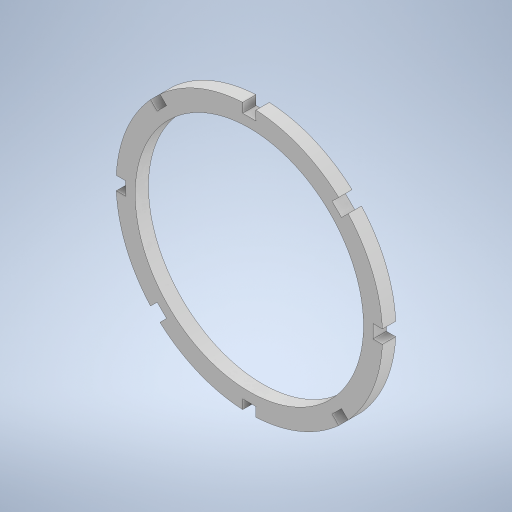
# Autodesk Inventor part: Ozji obroc
Saved by Autodesk Inventor 2023 (Build 270158000, 158)
## iProperties
Created: 2022-12-16
Part Number: Ozji obroc
Material: Generic
Document SubType Name: Modeling
Designer: David Zindović
Density: 1 g/cm^3
Appearance: Default
Author: David Zindović
Autodesk Inventor part; units mm, degrees
ref_plane "YZ Plane" through (0, 0, 0) normal (1, 0, 0) x (0, 1, 0)
ref_plane "XZ Plane" through (0, 0, 0) normal (0, 1, 0) x (-1, 0, 0)
ref_plane "XY Plane" through (0, 0, 0) normal (0, 0, 1) x (1, 0, 0)
sketch "Sketch1" plane through (0, 0, 0) normal (0, 0, 1) x (1, 0, 0)
  circle A0 centre (0, 0) radius 35
  circle A1 centre (0, 0) radius 30
  line L0 (32.5, 1.75) -> (35, 1.75)
  line L1 (35, 1.75) -> (35, -1.75)
  line L2 (35, -1.75) -> (32.5, -1.75)
  line L3 (32.5, -1.75) -> (32.5, 1.75)
  line L4 (30, 0) -> (35, 0)
  line L5 (24.2184, 21.7435) -> (21.7435, 24.2184)
  line L6 (21.7435, 24.2184) -> (23.5113, 25.9862)
  line L7 (25.9862, 23.5113) -> (24.2184, 21.7435)
  line L8 (23.5113, 25.9862) -> (25.9862, 23.5113)
  line L9 (1.75, 32.5) -> (-1.75, 32.5)
  line L10 (-1.75, 32.5) -> (-1.75, 35)
  line L11 (1.75, 35) -> (1.75, 32.5)
  line L12 (-1.75, 35) -> (1.75, 35)
  line L13 (-21.7435, 24.2184) -> (-24.2184, 21.7435)
  line L14 (-24.2184, 21.7435) -> (-25.9862, 23.5113)
  line L15 (-23.5113, 25.9862) -> (-21.7435, 24.2184)
  line L16 (-25.9862, 23.5113) -> (-23.5113, 25.9862)
  line L17 (-32.5, 1.75) -> (-32.5, -1.75)
  line L18 (-32.5, -1.75) -> (-35, -1.75)
  line L19 (-35, 1.75) -> (-32.5, 1.75)
  line L20 (-35, -1.75) -> (-35, 1.75)
  line L21 (-24.2184, -21.7435) -> (-21.7435, -24.2184)
  line L22 (-21.7435, -24.2184) -> (-23.5113, -25.9862)
  line L23 (-25.9862, -23.5113) -> (-24.2184, -21.7435)
  line L24 (-23.5113, -25.9862) -> (-25.9862, -23.5113)
  line L25 (-1.75, -32.5) -> (1.75, -32.5)
  line L26 (1.75, -32.5) -> (1.75, -35)
  line L27 (-1.75, -35) -> (-1.75, -32.5)
  line L28 (1.75, -35) -> (-1.75, -35)
  line L29 (21.7435, -24.2184) -> (24.2184, -21.7435)
  line L30 (24.2184, -21.7435) -> (25.9862, -23.5113)
  line L31 (23.5113, -25.9862) -> (21.7435, -24.2184)
  line L32 (25.9862, -23.5113) -> (23.5113, -25.9862)
  point P0 (32.5, 0)
  point P1 (32.5, 0)
  point P2 (22.981, 22.981)
  point P3 (0, 32.5)
  point P4 (-22.981, 22.981)
  point P5 (-32.5, 0)
  point P6 (-22.981, -22.981)
  point P7 (0, -32.5)
  point P8 (22.981, -22.981)
  point P9 (34.9562, 1.75)
  point P10 (25.9552, 23.4803)
  point P11 (23.4803, 25.9552)
  point P12 (1.75, 34.9562)
  point P13 (-1.75, 34.9562)
  point P14 (-23.4803, 25.9552)
  point P15 (-25.9552, 23.4803)
  point P16 (-34.9562, 1.75)
  point P17 (-34.9562, -1.75)
  point P18 (-25.9552, -23.4803)
  point P19 (-23.4803, -25.9552)
  point P20 (-1.75, -34.9562)
  point P21 (1.75, -34.9562)
  point P22 (23.4803, -25.9552)
  point P23 (25.9552, -23.4803)
  point P24 (34.9562, -1.75)
  dimension "d0" = 70
  dimension "d1" = 5
  dimension "d2" = 3.5
  dimension "d5" = 360
  constraints: 66 end point, 2 horizontal, 2 horizontal alignment, 2 midpoint, 2 parallel, 2 vertical alignment, 1 coincident, 1 perpendicular, 78 other
  measures "d2" distance of L2.end L0.start
extrude "Extrusion1" add sketch "Sketch1" along normal mid plane 3.5 contours L0 L3 L2 A0 L30 L29 L31 L26 L25 L27 L22 L21 L23 L18 L17 L19 L14 L13 L15 L10 L9 L11 L6 L5 L7
body "Solid1"
